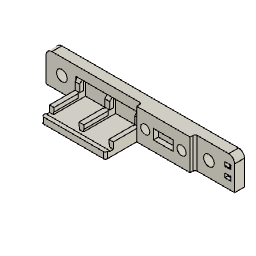
Bed WAGO Mount (Autodesk Fusion 360 design; units mm, degrees)
Autodesk Fusion 360 part; units mm, degrees
sketch "Sketch1" plane through (0, 0, 0) normal (0, 0, 1) x (1, 0, 0)
  line L0 (16.15, 6.1) -> (-16.15, 6.1)
  line L1 (-16.15, 6.1) -> (-16.15, -6.1)
  line L2 (-16.15, -6.1) -> (16.15, -6.1)
  line L3 (16.15, -6.1) -> (16.15, 6.1)
  line L4 (16.15, 6.1) -> (-16.15, -6.1) construction
  line L5 (-16.15, 6.1) -> (16.15, -6.1) construction
  dimension "d1" = 12.2
  dimension "d2" = 32.3
  constraint horizontal L0
  constraint perpendicular L0 L1
  constraint parallel L0 L2
  constraint parallel L1 L3
  constraint coincident L4 origin
  constraint coincident L5 origin
  measures "d1" distance of L0.start L2.end
  measures "d2" distance of L0.start L0.end
extrude "Extrude1" add sketch "Sketch1" along normal blind 22.25 makes body 1
sketch "Sketch2" plane through (0, 0, 22.25) normal (0, 0, 1) x (-1, 0, 0)
  line L0 (-16.15, 6.1) -> (-16.15, -6.1)
  line L1 (-16.15, -6.1) -> (16.15, -6.1)
  line L2 (16.15, -6.1) -> (16.15, 6.1)
  line L3 (16.15, 6.1) -> (-16.15, 6.1)
  line L4 (14.15, -6.1) -> (1, -6.1)
  line L5 (1, -6.1) -> (1, 4.1)
  line L6 (1, 4.1) -> (14.15, 4.1)
  line L7 (14.15, 4.1) -> (14.15, -6.1)
  line L8 (-1, -6.1) -> (-14.15, -6.1)
  line L9 (-14.15, -6.1) -> (-14.15, 4.1)
  line L10 (-14.15, 4.1) -> (-1, 4.1)
  line L11 (-1, 4.1) -> (-1, -6.1)
  dimension "d8" = 2
  dimension "d11" = 2
  dimension "d48" = 2
  dimension "d52" = 2
  constraint horizontal L4
  constraint vertical L5
  constraint horizontal L6
  constraint vertical L7
  constraint coincident L1 L4.start
  constraint horizontal L8
  constraint vertical L9
  constraint horizontal L10
  constraint vertical L11
  constraint coincident L1 L8.start
  constraint equal L6 L10
  constraint equal L5 L11
  measures "d8" distance of L4.end L8.start
  measures "d11" distance of L3 L9.end
  measures "d48" distance of L1.end L4.start
  measures "d52" distance of L0.end L8.end
extrude "Extrude2" cut sketch "Sketch2" against normal blind 20.25 contours L1 L8 L9 L10 L11 | L1 L4 L5 L6 L7 bodies 1
sketch "Sketch3" plane through (0, 0, 2) normal (0, 0, 1) x (-1, 0, 0)
  line L0 (-1, 4.1) -> (-14.15, 4.1)
  line L1 (-14.15, -6.1) -> (-1, -6.1)
  line L2 (-1, -6.1) -> (-1, 4.1)
  line L3 (14.15, 4.1) -> (1, 4.1)
  line L4 (1, 4.1) -> (1, -6.1)
  line L5 (1, -6.1) -> (14.15, -6.1)
  line L6 (14.15, -6.1) -> (14.15, 4.1)
  line L7 (-14.15, -6.1) -> (-1, -6.1)
  line L8 (-1, -6.1) -> (-14.15, -6.1)
  line L9 (-14.15, -6.1) -> (-14.15, -4.1)
  line L10 (-14.15, -4.1) -> (-1, -4.1)
  line L11 (-1, -4.1) -> (-1, -6.1)
  line L12 (-1, 4.1) -> (-14.15, 4.1)
  line L13 (-1, -6.1) -> (-1, 4.1)
  line L14 (14.15, 4.1) -> (1, 4.1)
  line L15 (1, 4.1) -> (1, -6.1)
  line L16 (1, -6.1) -> (14.15, -6.1)
  line L17 (14.15, -6.1) -> (14.15, 4.1)
  line L18 (1, -4.1) -> (14.15, -4.1)
  line L19 (-14.15, 4.1) -> (-14.15, -6.1)
  line L20 (-14.15, 4.1) -> (-14.15, -6.1)
  dimension "d12" = 2
  constraint horizontal L8
  constraint vertical L9
  constraint horizontal L10
  constraint vertical L11
  constraint coincident L1.end L2.start
  constraint coincident L15 L18.start
  constraint coincident L17 L18.end
  constraint perpendicular L17 L18
  constraint collinear L10 L18
  constraint coincident L1.start L7.start
  measures "d12" distance of L1.start L9.end
extrude "Extrude3" add sketch "Sketch3" along normal blind 2 contours L1 L2 L7 L8 L9 L10 L11 L13 L19 L20 | L4 L5 L6 L15 L16 L17 L18 bodies 1
sketch "Sketch4" plane through (0, 0, 22.25) normal (0, 0, 1) x (-1, 0, 0)
  line L0 (-1, 4.1) -> (-1, -6.1)
  line L1 (-1, -6.1) -> (1, -6.1)
  line L2 (1, -6.1) -> (1, 4.1)
  line L3 (1, 4.1) -> (14.15, 4.1)
  line L4 (14.15, 4.1) -> (14.15, -6.1)
  line L5 (14.15, -6.1) -> (16.15, -6.1)
  line L6 (16.15, -6.1) -> (16.15, 6.1)
  line L7 (16.15, 6.1) -> (-16.15, 6.1)
  line L8 (-16.15, 6.1) -> (-16.15, -6.1)
  line L9 (-14.15, 4.1) -> (-1, 4.1)
  line L10 (16.15, 4.1) -> (-16.15, 4.1)
  line L11 (-16.15, -6.1) -> (-14.15, -6.1)
  line L12 (-14.15, -6.1) -> (-14.15, 4.1)
  constraint coincident L6 L10.start
  constraint coincident L8 L10.end
  constraint perpendicular L8 L10
extrude "Extrude4" cut sketch "Sketch4" against normal blind 4 contours L0 L1 L2 L10 | L8 L10 L11 L12 | L4 L5 L6 L10 bodies 1
sketch "Sketch5" plane through (0, 0, 18.25) normal (0, 0, 1) x (-1, 0, 0)
  line L0 (16.15, 4.1) -> (14.15, 4.1)
  line L1 (14.15, 4.1) -> (14.15, -6.1)
  line L2 (-14.15, 4.1) -> (-16.15, 4.1)
  line L3 (-16.15, 4.1) -> (-16.15, -6.1)
  line L4 (-16.15, -6.1) -> (-14.15, -6.1)
  line L5 (1, -6.1) -> (1, 4.1)
  line L6 (1, 4.1) -> (-1, 4.1)
  line L7 (-1, 4.1) -> (-1, -6.1)
  line L8 (-1, -6.1) -> (1, -6.1)
  line L9 (16.15, 4.1) -> (14.15, 4.1)
  line L10 (16.15, -6.1) -> (16.15, 4.1)
  line L11 (16.15, -6.1) -> (-16.15, -6.1)
  line L12 (-16.15, -6.1) -> (-16.15, 0.85)
  line L13 (-16.15, 0.85) -> (16.15, 0.85)
  line L14 (16.15, 0.85) -> (16.15, -6.1)
  line L15 (16.15, -6.1) -> (16.15, 4.1)
  line L16 (14.15, 4.1) -> (14.15, -6.1)
  line L17 (14.15, -6.1) -> (16.15, -6.1)
  line L18 (14.15, -6.1) -> (16.15, -6.1)
  line L19 (-14.15, -6.1) -> (-14.15, 4.1)
  dimension "d17" = 3.25
  constraint horizontal L11
  constraint vertical L12
  constraint horizontal L13
  constraint vertical L14
  constraint coincident L3 L12.end
  constraint coincident L3.end L4.start
  constraint coincident L10.start L11.start
  measures "d17" distance of L2.end L12.end
extrude "Extrude5" cut sketch "Sketch5" against normal blind 13 contours L1 L10 L11 L13 L14 L15 L16 L17 L18 | L1 L5 L11 L13 L16 | L5 L7 L8 L11 L13 | L7 L11 L13 L19 | L3 L4 L11 L12 L13 L19 bodies 1
sketch "Sketch6" plane through (0, 0, 22.25) normal (0, 0, 1) x (-1, 0, 0)
  line L0 (-16.15, 4.1) -> (16.15, 4.1)
  line L1 (16.15, 4.1) -> (16.15, 6.1)
  line L2 (16.15, 6.1) -> (-16.15, 6.1)
  line L3 (-16.15, 6.1) -> (-16.15, 4.1)
  line L4 (16.15, 6.1) -> (-16.15, 6.1)
  line L5 (-16.15, 6.1) -> (-16.15, 3.6)
  line L6 (-16.15, 3.6) -> (16.15, 3.6)
  line L7 (16.15, 3.6) -> (16.15, 6.1)
  dimension "d20" = 2.5
  constraint horizontal L4
  constraint vertical L5
  constraint horizontal L6
  constraint vertical L7
  constraint coincident L1.end L2.start
  constraint collinear L3 L5
  measures "d20" distance of L2.end L5.end
extrude "Extrude6" add sketch "Sketch6" against normal blind 2 contours L0 L5 L6 L7 bodies 1
sketch "Sketch7" plane through (0, 0, 18.25) normal (0, 0, 1) x (-1, 0, 0)
  line L0 (16.15, 4.1) -> (14.15, 4.1)
  line L1 (14.15, 4.1) -> (14.15, 0.85) construction
  line L2 (13.9, 2.85) -> (16.15, 2.85)
  line L3 (1.25, 0.85) -> (-1.25, 0.85)
  line L4 (-1.25, 0.85) -> (-1.25, 2.85)
  line L5 (-1.25, 2.85) -> (1.25, 2.85)
  line L6 (1.25, 2.85) -> (1.25, 0.85)
  line L7 (16.15, 0.85) -> (13.9, 0.85)
  line L8 (13.9, 0.85) -> (13.9, 2.85)
  line L9 (13.9, 2.85) -> (16.15, 2.85)
  line L10 (16.15, 2.85) -> (16.15, 0.85)
  line L11 (-13.9, 0.85) -> (-16.15, 0.85)
  line L12 (-16.15, 0.85) -> (-16.15, 2.85)
  line L13 (-16.15, 2.85) -> (-13.9, 2.85)
  line L14 (-13.9, 2.85) -> (-13.9, 0.85)
  line L15 (16.15, 0.85) -> (16.15, 4.1)
  line L16 (16.15, 4.1) -> (14.15, 4.1)
  line L17 (1, 0.85) -> (1, 4.1) construction
  line L18 (1, 4.1) -> (-1, 4.1)
  line L19 (-1, 4.1) -> (-1, 0.85) construction
  line L20 (-16.15, 0.85) -> (-14.15, 0.85)
  line L21 (-14.15, 4.1) -> (-16.15, 4.1)
  line L22 (-16.15, 4.1) -> (-16.15, 0.85)
  line L23 (16.15, 0.85) -> (16.15, 4.1)
  line L24 (14.15, 4.1) -> (14.15, 0.85)
  line L25 (14.15, 0.85) -> (16.15, 0.85)
  line L26 (14.15, 0.85) -> (16.15, 0.85)
  line L27 (-1, 0.85) -> (1, 0.85)
  line L28 (-14.15, 0.85) -> (-14.15, 4.1)
  dimension "d23" = 2.25
  dimension "d50" = 2
  dimension "d51" = 2.5
  constraint horizontal L2
  constraint horizontal L3
  constraint vertical L4
  constraint horizontal L5
  constraint vertical L6
  constraint horizontal L7
  constraint vertical L8
  constraint horizontal L9
  constraint vertical L10
  constraint horizontal L11
  constraint vertical L12
  constraint horizontal L13
  constraint vertical L14
  constraint equal L7 L11
  constraint equal L4 L14
  constraint coincident L7.start L10.end
  constraint coincident L11.end L12.start
  constraint equal L6 L8
  measures "d23" distance of L7.start L7.end
  measures "d50" distance of L3.start L5.end
  measures "d51" distance of L3.start L3.end
extrude "Extrude7" add sketch "Sketch7" against normal blind 12.25 contours L2 L7 L9 L10 L15 L23 L24 L25 L26 | L2 L7 L8 L9 L24 | L3 L4 L5 L6 L27 | L11 L13 L14 L28 | L11 L12 L13 L20 L22 L28 bodies 1
sketch "Sketch8" plane through (0, 0, 5.25) normal (0, 0, 1) x (-1, 0, 0)
  line L0 (14.15, -6.1) -> (16.15, -6.1) construction
  line L1 (14.15, -6.1) -> (16.15, -6.1) construction
  line L2 (-14.15, 0.85) -> (-16.15, 0.85) construction
  line L3 (-16.15, 0.85) -> (-16.15, -6.1) construction
  line L4 (-16.15, -6.1) -> (-14.15, -6.1) construction
  line L5 (-1, -6.1) -> (-1, -4.1) construction
  line L6 (-1, -4.1) -> (-14.15, -4.1) construction
  line L7 (-14.15, -6.1) -> (-1, -6.1) construction
  line L8 (16.15, -6.1) -> (-16.15, -6.1)
  line L9 (-16.15, -6.1) -> (-16.15, -4.1)
  line L10 (-16.15, -4.1) -> (16.15, -4.1)
  line L11 (16.15, -4.1) -> (16.15, -6.1)
  line L12 (16.15, 0.85) -> (14.15, 0.85)
  line L13 (16.15, 0.85) -> (14.15, 0.85)
  line L14 (14.15, 0.85) -> (14.15, -6.1)
  line L15 (16.15, -6.1) -> (16.15, 0.85)
  line L16 (14.15, 0.85) -> (14.15, -6.1)
  line L17 (16.15, -6.1) -> (16.15, 0.85)
  line L18 (-14.15, -6.1) -> (-14.15, 0.85)
  line L19 (-14.15, -4.1) -> (-14.15, -6.1)
  constraint horizontal L8
  constraint vertical L9
  constraint horizontal L10
  constraint vertical L11
  constraint coincident L3 L9.end
  constraint coincident L0.end L1.end
  constraint coincident L6.end L10
extrude "Extrude8" cut sketch "Sketch8" against normal up to surface (1.25 mm away) contours L8 L10 L11 L14 L15 L16 L17 | L8 L10 L14 L16 L18 L19 | L8 L9 L10 L18 L19 bodies 1
sketch "Sketch9" plane through (0, 0, 5.25) normal (0, 0, 1) x (-1, 0, 0)
  line L0 (14.15, -4.1) -> (16.15, -4.1)
  line L1 (-16.15, -6.1) -> (16.15, -6.1)
  line L2 (16.15, -4.1) -> (14.15, -4.1)
  line L3 (-1, -4.1) -> (-14.15, -4.1)
  line L4 (16.15, -4.1) -> (13.9, -4.1)
  line L5 (13.9, -4.1) -> (13.9, 0.85)
  line L6 (13.9, 0.85) -> (16.15, 0.85)
  line L7 (16.15, 0.85) -> (16.15, -4.1)
  line L8 (1.25, -4.1044) -> (-1.25, -4.1044)
  line L9 (-1.25, -4.1044) -> (-1.25, 0.85)
  line L10 (-1.25, 0.85) -> (1.25, 0.85)
  line L11 (1.25, 0.85) -> (1.25, -4.1044)
  line L12 (-16.15, -4.1) -> (-13.9, -4.1)
  line L13 (-13.9, -4.1) -> (-13.9, 0.8544)
  line L14 (-13.9, 0.8544) -> (-16.15, 0.8544)
  line L15 (-16.15, 0.8544) -> (-16.15, -4.1)
  line L16 (16.15, 4.1) -> (14.15, 4.1)
  line L17 (14.15, 4.1) -> (14.15, 2.85)
  line L18 (13.9, 0.85) -> (16.15, 0.85)
  line L19 (14.15, -4.1) -> (1, -4.1)
  line L20 (16.15, 0.85) -> (16.15, 4.1)
  line L21 (14.15, 2.85) -> (13.9, 2.85)
  line L22 (13.9, 2.85) -> (13.9, 0.85)
  line L23 (1, 4.1) -> (-1, 4.1)
  line L24 (-1, 4.1) -> (-1, 2.85)
  line L25 (-1, 2.85) -> (-1.25, 2.85)
  line L26 (-1.25, 2.85) -> (-1.25, 0.85)
  line L27 (-1.25, 0.85) -> (1.25, 0.85)
  line L28 (1.25, 0.85) -> (1.25, 2.85)
  line L29 (16.15, 0.85) -> (14.15, 0.85)
  line L30 (13.9, 0.85) -> (16.15, 0.85)
  line L31 (16.15, -4.1) -> (16.15, 0.85)
  line L32 (14.15, 0.85) -> (14.15, -4.1)
  line L33 (16.15, -6.1) -> (16.15, -4.1)
  line L34 (1, -4.1) -> (-1, -4.1)
  line L35 (-14.15, -4.1) -> (-16.15, -4.1)
  line L36 (-16.15, -4.1) -> (-16.15, -6.1)
  line L37 (1, 2.85) -> (1, 4.1)
  line L38 (1.25, 2.85) -> (1, 2.85)
  line L39 (-14.15, 2.85) -> (-14.15, 4.1)
  line L40 (-14.15, 4.1) -> (-16.15, 4.1)
  line L41 (-16.15, 4.1) -> (-16.15, 0.85)
  line L42 (-16.15, 0.85) -> (-13.9, 0.85)
  line L43 (-13.9, 0.85) -> (-13.9, 2.85)
  line L44 (-13.9, 2.85) -> (-14.15, 2.85)
  constraint horizontal L4
  constraint vertical L5
  constraint horizontal L6
  constraint vertical L7
  constraint coincident L0.end L2.start
  constraint horizontal L8
  constraint vertical L9
  constraint horizontal L10
  constraint vertical L11
  constraint horizontal L12
  constraint vertical L13
  constraint horizontal L14
  constraint vertical L15
  constraint equal L9 L13
  constraint equal L6 L14
  constraint equal L6 L18
  constraint coincident L5.end L6.start
  constraint coincident L10.end L11.start
  constraint coincident L12.start L15.end
  constraint coincident L9.end L10.start
extrude "Extrude9" add sketch "Sketch9" against normal blind 2 contours L0 L2 L4 L6 L7 L18 L29 L30 L31 L32 | L4 L5 L6 L18 L19 L30 L32 | L3 L9 L10 L11 L19 L27 L34 | L3 L8 L9 L11 L19 L34 | L3 L12 L13 L15 L35 L42 | L13 L14 L15 L41 L42 L43 bodies 1
chamfer "Chamfer1" distance 1.25 angle 45 5 edges at (-15.025, 4.1, 5.25) (-15.025, 4.1, 5.25) (15.025, 4.1, 5.25) (0, 4.1044, 5.25) (15.025, 4.1, 5.25) on bodies 1
move_body "Move1" bodies 1 to x (1, 0, 0) y (0, 0, 1) z (0, -1, 0) at (0, 0, 0)
extrude "Extrude22" add 1 faces at (-5.3833, -7.4167, -6.1) along direction (0, 0, -1) blind 1 on bodies 1 bodies 1
sketch "Sketch10" plane through (0, 0, 0) normal (0, 1, 0) x (-1, 0, 0)
  line L0 (42.15, -7.1) -> (58.15, -7.1)
  line L1 (58.15, -7.1) -> (58.15, 8.9)
  line L2 (58.15, 8.9) -> (42.15, 8.9)
  line L3 (42.15, 8.9) -> (42.15, -7.1)
  line L4 (-16.15, -7.1) -> (-32.15, -7.1)
  line L5 (-32.15, -7.1) -> (-32.15, 8.9)
  line L6 (-32.15, 8.9) -> (-16.15, 8.9)
  line L7 (-16.15, 8.9) -> (-16.15, -7.1)
  line L8 (42.15, 8.9) -> (58.15, -7.1) construction
  line L9 (-32.15, -7.1) -> (-16.15, 8.9) construction
  circle A0 centre (50.15, 0.9) radius 2.7
  circle A1 centre (-24.15, 0.9) radius 2.7
  line L10 (-16.15, 6.1) -> (-16.15, -7.1)
  line L11 (16.15, -7.1) -> (16.15, 6.1)
  line L12 (16.15, 6.1) -> (-16.15, 6.1)
  line L13 (16.15, -7.1) -> (42.15, -7.1)
  line L14 (42.15, 8.9) -> (-16.15, 8.9)
  line L15 (-16.15, -7.1) -> (16.15, -7.1)
  dimension "d35" = 5.4
  dimension "d55" = 16
  dimension "d72" = 26
  constraint horizontal L0
  constraint vertical L1
  constraint horizontal L2
  constraint vertical L3
  constraint horizontal L4
  constraint vertical L5
  constraint horizontal L6
  constraint vertical L7
  constraint equal L1 L5
  constraint equal L1 L2
  constraint equal L5 L6
  constraint midpoint L8 A0.centre
  constraint midpoint L9 A1.centre
  constraint equal A0 A1
  constraint coincident L4.start L7.end
  constraint coincident L11.start L13.start
  constraint perpendicular L11 L13
  constraint coincident L0.start L3.end
  measures "d35" diameter of A0
  measures "d55" distance of L0.end L1.end
  measures "d72" distance of L11.start L0.start
extrude "Extrude10" add sketch "Sketch10" against normal blind 4 contours L0 L1 L2 L3 | L3 L7 L11 L12 L13 L14 | L4 L5 L6 L7 L10 bodies 1
extrude "Extrude17" add 1 faces at (-1.0667, 0, -5.2128) along direction (0, 1, 0) blind 1 on bodies 1 bodies 1
sketch "Sketch19" plane through (0, -4, 0) normal (0, -1, 0) x (1, 0, 0)
  line L0 (-29.65, 4.9) -> (-29.65, -3.1) construction
  line L1 (-38.85, 0.9) -> (-20.45, 0.9) construction
  circle A0 centre (-38.85, 0.9) radius 2.3
  circle A1 centre (-20.45, 0.9) radius 2.3
  circle A2 centre (24.15, 0.9) radius 2.7
  circle A3 centre (-50.15, 0.9) radius 2.7
  line L2 (-1.25, 4.1) -> (-1.25, 4.1044)
  line L3 (-1.25, 4.1044) -> (1.25, 4.1044)
  line L4 (1.25, 4.1044) -> (1.25, 4.1)
  line L5 (1.25, 4.1) -> (13.9, 4.1)
  line L6 (13.9, 4.1) -> (16.15, 4.1)
  line L7 (16.15, 4.1) -> (16.15, -7.1)
  line L8 (16.15, -7.1) -> (32.15, -7.1)
  line L9 (32.15, -7.1) -> (32.15, 8.9)
  line L10 (32.15, 8.9) -> (-58.15, 8.9)
  line L11 (-58.15, 8.9) -> (-58.15, -7.1)
  line L12 (-58.15, -7.1) -> (-16.15, -7.1)
  line L13 (-16.15, -7.1) -> (-16.15, 4.1)
  line L14 (-16.15, 4.1) -> (-13.9, 4.1)
  line L15 (-13.9, 4.1) -> (-1.25, 4.1)
  line L16 (-42.15, 4.9) -> (-17.15, 4.9) construction
  line L17 (-17.15, 4.9) -> (-17.15, -3.1) construction
  line L18 (-17.15, -3.1) -> (-42.15, -3.1) construction
  line L19 (-42.15, -3.1) -> (-42.15, 4.9) construction
  line L20 (-42.15, 0.9) -> (-58.15, 0.9) construction
  dimension "d91" = 18.4
  dimension "d92" = 4.6
  dimension "d93" = 4.6
  dimension "d97" = 8
  dimension "d98" = 25
  dimension "d108" = 1
  constraint horizontal L1
  constraint midpoint L0 L1
  constraint coincident L1.start A0.centre
  constraint coincident L1.end A1.centre
  constraint horizontal L16
  constraint vertical L17
  constraint horizontal L18
  constraint vertical L19
  constraint midpoint L19 L20.start
  constraint perpendicular L19 L20
  constraint midpoint L11 L20.end
  constraint midpoint L0.start L16
  constraint midpoint L0.end L18
  measures "d91" distance of L1.start L1.end
  measures "d92" diameter of A0
  measures "d93" diameter of A1
  measures "d97" distance of L16.start L18.end
  measures "d98" distance of L16.start L16.end
  measures "d108" distance of L13 L17
extrude "Extrude20" cut sketch "Sketch19" against normal blind 4 contours A0 | A1 bodies 1
sketch "Sketch21" plane through (0, -4, 0) normal (0, -1, 0) x (1, 0, 0)
  circle A0 centre (-20.45, 0.9) radius 2.3
  circle A1 centre (-38.85, 0.9) radius 2.3
  circle A2 centre (24.15, 0.9) radius 2.7
  circle A3 centre (-50.15, 0.9) radius 2.7
  line L0 (-1.25, 4.1) -> (-1.25, 4.1044)
  line L1 (-1.25, 4.1044) -> (1.25, 4.1044)
  line L2 (1.25, 4.1044) -> (1.25, 4.1)
  line L3 (1.25, 4.1) -> (13.9, 4.1)
  line L4 (13.9, 4.1) -> (16.15, 4.1)
  line L5 (16.15, 4.1) -> (16.15, -7.1)
  line L6 (16.15, -7.1) -> (32.15, -7.1)
  line L7 (32.15, -7.1) -> (32.15, 8.9)
  line L8 (32.15, 8.9) -> (-58.15, 8.9)
  line L9 (-58.15, 8.9) -> (-58.15, -7.1)
  line L10 (-58.15, -7.1) -> (-16.15, -7.1)
  line L11 (-16.15, -7.1) -> (-16.15, 4.1)
  line L12 (-16.15, 4.1) -> (-13.9, 4.1)
  line L13 (-13.9, 4.1) -> (-1.25, 4.1)
  line L14 (-34.65, 3.4) -> (-24.65, 3.4)
  line L15 (-24.65, 3.4) -> (-24.65, -1.6)
  line L16 (-24.65, -1.6) -> (-34.65, -1.6)
  line L17 (-34.65, -1.6) -> (-34.65, 3.4)
  line L18 (-38.85, 0.9) -> (-34.65, 0.9) construction
  line L19 (-24.65, 0.9) -> (-20.45, 0.9) construction
  dimension "d99" = 10
  dimension "d100" = 5
  constraint horizontal L14
  constraint vertical L15
  constraint horizontal L16
  constraint vertical L17
  constraint coincident A1.centre L18.start
  constraint perpendicular L17 L18
  constraint midpoint L17 L18.end
  constraint midpoint L15 L19.start
  constraint perpendicular L15 L19
  constraint coincident A0.centre L19.end
  constraint equal L18 L19
  measures "d99" distance of L14.start L14.end
  measures "d100" distance of L14.start L16.end
extrude "Extrude21" cut sketch "Sketch21" against normal blind 2.5 contours L14 L15 L16 L17 bodies 1
sketch "Sketch11" plane through (0, -4, 0) normal (0, -1, 0) x (1, 0, 0)
  circle A0 centre (24.15, 0.9) radius 6
  circle A1 centre (-50.15, 0.9) radius 6
  circle A2 centre (24.15, 0.9) radius 2.7
  circle A3 centre (-50.15, 0.9) radius 2.7
  line L0 (-1.25, 4.1) -> (-1.25, 4.1044)
  line L1 (-1.25, 4.1044) -> (1.25, 4.1044)
  line L2 (1.25, 4.1044) -> (1.25, 4.1)
  line L3 (1.25, 4.1) -> (13.9, 4.1)
  line L4 (13.9, 4.1) -> (16.15, 4.1)
  line L5 (16.15, 4.1) -> (16.15, -7.1)
  line L6 (16.15, -7.1) -> (32.15, -7.1)
  line L7 (32.15, -7.1) -> (32.15, 8.9)
  line L8 (32.15, 8.9) -> (-58.15, 8.9)
  line L9 (-58.15, 8.9) -> (-58.15, -7.1)
  line L10 (-16.15, -7.1) -> (-16.15, 4.1)
  line L11 (-16.15, 4.1) -> (-13.9, 4.1)
  line L12 (-13.9, 4.1) -> (-1.25, 4.1)
  line L13 (-58.15, -7.1) -> (-16.15, -7.1)
  line L14 (-24.65, 3.4) -> (-24.65, -1.6)
  line L15 (-24.65, -1.6) -> (-34.65, -1.6)
  line L16 (-34.65, -1.6) -> (-34.65, 3.4)
  line L17 (-34.65, 3.4) -> (-24.65, 3.4)
  circle A4 centre (-20.45, 0.9) radius 2.3
  circle A5 centre (-38.85, 0.9) radius 2.3
  dimension "d38" = 12
  dimension "d39" = 12
  constraint coincident A0.centre A2.centre
  constraint coincident A1.centre A3.centre
  measures "d38" diameter of A0
  measures "d39" diameter of A1
extrude "Extrude11" [suppressed]
sketch "Sketch13" plane through (0, 1, 0) normal (0, 1, 0) x (-1, 0, 0)
  line L0 (33, 2.9) -> (-7, 2.9)
  line L1 (-7, 2.9) -> (-7, -1.1)
  line L2 (-7, -1.1) -> (33, -1.1)
  line L3 (33, -1.1) -> (33, 2.9)
  line L4 (-7, 0.9) -> (-24.15, 0.9) construction
  line L5 (33, 0.9) -> (50.15, 0.9) construction
  circle A0 centre (50.15, 0.9) radius 2.7
  circle A1 centre (-24.15, 0.9) radius 2.7
  dimension "d61" = 4
  dimension "d62" = 40
  constraint horizontal L0
  constraint perpendicular L0 L1
  constraint parallel L0 L2
  constraint parallel L1 L3
  constraint midpoint L1 L4.start
  constraint perpendicular L1 L4
  constraint midpoint L3 L5.start
  constraint perpendicular L3 L5
  constraint coincident L4.end A1.centre
  constraint coincident L5.end A0.centre
  constraint equal L4 L5
  measures "d61" distance of L0.start L2.end
  measures "d62" distance of L0.start L0.end
extrude "Extrude15" add sketch "Sketch13" along normal blind 0.8 contours L0 L1 L2 L3 bodies 1
sketch "Sketch22" plane through (0, -4, 0) normal (0, -1, 0) x (1, 0, 0)
  line L0 (-24.65, 3.4) -> (-24.65, -1.6)
  line L1 (-24.65, -1.6) -> (-34.65, -1.6)
  line L2 (-34.65, -1.6) -> (-34.65, 3.4)
  line L3 (-34.65, 3.4) -> (-24.65, 3.4)
  circle A0 centre (-20.45, 0.9) radius 2.3
  circle A1 centre (-38.85, 0.9) radius 2.3
  line L4 (-1.25, 4.1) -> (-1.25, 4.1044)
  line L5 (-1.25, 4.1044) -> (1.25, 4.1044)
  line L6 (1.25, 4.1044) -> (1.25, 4.1)
  line L7 (1.25, 4.1) -> (13.9, 4.1)
  line L8 (13.9, 4.1) -> (16.15, 4.1)
  line L9 (16.15, 4.1) -> (16.15, -7.1)
  line L10 (16.15, -7.1) -> (32.15, -7.1)
  line L11 (32.15, -7.1) -> (32.15, 8.9)
  line L12 (32.15, 8.9) -> (-58.15, 8.9)
  line L13 (-58.15, 8.9) -> (-58.15, -7.1)
  line L14 (-58.15, -7.1) -> (-16.15, -7.1)
  line L15 (-16.15, -7.1) -> (-16.15, 4.1)
  line L16 (-16.15, 4.1) -> (-13.9, 4.1)
  line L17 (-13.9, 4.1) -> (-1.25, 4.1)
  line L18 (-58.15, 8.9) -> (-63.15, 8.9)
  line L19 (-63.15, 8.9) -> (-63.15, -7.1)
  line L20 (-63.15, -7.1) -> (-58.15, -7.1)
  line L21 (-61.15, 4.4) -> (-58.15, 4.4)
  line L22 (-58.15, 4.4) -> (-58.15, 2.4)
  line L23 (-58.15, 2.4) -> (-61.15, 2.4)
  line L24 (-61.15, 2.4) -> (-61.15, 4.4)
  line L25 (-61.15, -0.6) -> (-58.15, -0.6)
  line L26 (-58.15, -0.6) -> (-58.15, -2.6)
  line L27 (-58.15, -2.6) -> (-61.15, -2.6)
  line L28 (-61.15, -2.6) -> (-61.15, -0.6)
  line L29 (-61.15, 2.4) -> (-61.15, -0.6) construction
  line L30 (-61.15, 0.9) -> (-63.15, 0.9) construction
  circle A2 centre (-50.15, 0.9) radius 2.7
  circle A3 centre (24.15, 0.9) radius 2.7
  dimension "d115" = 3
  dimension "d116" = 2
  dimension "d117" = 5
  dimension "d118" = 3
  constraint coincident L12.end L13.start
  constraint perpendicular L13 L18
  constraint perpendicular L14 L19
  constraint coincident L13.end L14.start
  constraint perpendicular L13 L20
  constraint horizontal L21
  constraint vertical L22
  constraint horizontal L23
  constraint vertical L24
  constraint horizontal L25
  constraint vertical L26
  constraint horizontal L27
  constraint vertical L28
  constraint equal L24 L28
  constraint equal L21 L25
  constraint perpendicular L23 L29
  constraint coincident L25.start L28.end
  constraint collinear L13 L22
  constraint midpoint L29 L30.start
  constraint perpendicular L29 L30
  constraint midpoint L19 L30.end
  measures "d115" distance of L21.start L21.end
  measures "d116" distance of L21.start L23.end
  measures "d117" distance of L12.end L18.end
  measures "d118" distance of L23.end L25.start
extrude "Extrude24" add sketch "Sketch22" against normal up to surface (5 mm away) contours L13 L18 L19 L20 L21 L23 L24 L25 L27 L28 bodies 1
sketch "Sketch23" plane through (0, 1, 0) normal (0, 1, 0) x (-1, 0, 0)
  line L0 (63.15, 8.9) -> (-32.15, 8.9)
  line L1 (-32.15, 8.9) -> (-32.15, -7.1)
  line L2 (-32.15, -7.1) -> (63.15, -7.1)
  line L3 (63.15, -7.1) -> (63.15, 8.9)
  line L4 (58.15, -2.6) -> (58.15, -0.6)
  line L5 (58.15, -0.6) -> (61.15, -0.6)
  line L6 (61.15, -0.6) -> (61.15, -2.6)
  line L7 (61.15, -2.6) -> (58.15, -2.6)
  line L8 (33, -1.1) -> (-7, -1.1)
  line L9 (-7, -1.1) -> (-7, 2.9)
  line L10 (-7, 2.9) -> (33, 2.9)
  line L11 (33, 2.9) -> (33, -1.1)
  circle A0 centre (50.15, 0.9) radius 2.7
  circle A1 centre (-24.15, 0.9) radius 2.7
  line L12 (58.15, 4.4) -> (61.15, 4.4)
  line L13 (61.15, 4.4) -> (61.15, 2.4)
  line L14 (61.15, 2.4) -> (58.15, 2.4)
  line L15 (58.15, 2.4) -> (58.15, 4.4)
  line L16 (58.15, 2.4) -> (58.15, -0.6)
  line L17 (61.15, 2.4) -> (61.15, -0.6)
  constraint coincident L14.end L15.start
  constraint coincident L4.end L5.start
  constraint coincident L13.end L14.start
  constraint coincident L5.end L6.start
extrude "Extrude25" cut sketch "Sketch23" against normal up to surface (4 mm away) contours L5 L14 L16 L17 bodies 1
sketch "Sketch24" plane through (0, 1, 0) normal (0, 1, 0) x (-1, 0, 0)
  line L0 (58.15, -2.6) -> (58.15, 4.4)
  line L1 (58.15, 4.4) -> (61.15, 4.4)
  line L2 (61.15, 4.4) -> (61.15, -2.6)
  line L3 (61.15, -2.6) -> (58.15, -2.6)
  line L4 (63.15, 8.9) -> (-32.15, 8.9)
  line L5 (-32.15, 8.9) -> (-32.15, -7.1)
  line L6 (-32.15, -7.1) -> (63.15, -7.1)
  line L7 (63.15, -7.1) -> (63.15, 8.9)
  line L8 (33, -1.1) -> (-7, -1.1)
  line L9 (-7, -1.1) -> (-7, 2.9)
  line L10 (-7, 2.9) -> (33, 2.9)
  line L11 (33, 2.9) -> (33, -1.1)
  circle A0 centre (50.15, 0.9) radius 2.7
  circle A1 centre (-24.15, 0.9) radius 2.7
extrude "Extrude26" add sketch "Sketch24" against normal up to surface (2.5 mm away) contours L0 L1 L2 L3 bodies 1
sketch "Sketch25" plane through (0, -4, 0) normal (0, -1, 0) x (1, 0, 0)
  line L0 (-58.15, 4.4) -> (-58.15, 2.4)
  line L1 (-58.15, 2.4) -> (-61.15, 2.4)
  line L2 (-61.15, 2.4) -> (-61.15, 4.4)
  line L3 (-61.15, 4.4) -> (-58.15, 4.4)
  line L4 (32.15, 8.9) -> (-63.15, 8.9)
  line L5 (-63.15, 8.9) -> (-63.15, -7.1)
  line L6 (-63.15, -7.1) -> (-16.15, -7.1)
  line L7 (-16.15, -7.1) -> (-16.15, 4.1)
  line L8 (-16.15, 4.1) -> (-13.9, 4.1)
  line L9 (-13.9, 4.1) -> (-1.25, 4.1)
  line L10 (-1.25, 4.1) -> (-1.25, 4.1044)
  line L11 (-1.25, 4.1044) -> (1.25, 4.1044)
  line L12 (1.25, 4.1044) -> (1.25, 4.1)
  line L13 (1.25, 4.1) -> (13.9, 4.1)
  line L14 (13.9, 4.1) -> (16.15, 4.1)
  line L15 (16.15, 4.1) -> (16.15, -7.1)
  line L16 (16.15, -7.1) -> (32.15, -7.1)
  line L17 (32.15, -7.1) -> (32.15, 8.9)
  line L18 (-24.65, 3.4) -> (-24.65, -1.6)
  line L19 (-24.65, -1.6) -> (-34.65, -1.6)
  line L20 (-34.65, -1.6) -> (-34.65, 3.4)
  line L21 (-34.65, 3.4) -> (-24.65, 3.4)
  circle A0 centre (-20.45, 0.9) radius 2.3
  circle A1 centre (-38.85, 0.9) radius 2.3
  line L22 (-58.15, -2.6) -> (-61.15, -2.6)
  line L23 (-61.15, -2.6) -> (-61.15, -0.6)
  line L24 (-61.15, -0.6) -> (-58.15, -0.6)
  line L25 (-58.15, -0.6) -> (-58.15, -2.6)
  line L26 (-43.15, 8.9) -> (-16.15, 8.9)
  line L27 (-16.15, 8.9) -> (-16.15, -7.1)
  line L28 (-16.15, -7.1) -> (-43.15, -7.1)
  line L29 (-43.15, -7.1) -> (-43.15, 8.9)
  circle A2 centre (-50.15, 0.9) radius 2.7
  circle A3 centre (24.15, 0.9) radius 2.7
  dimension "d131" = 27
  constraint horizontal L26
  constraint vertical L27
  constraint horizontal L28
  constraint vertical L29
  constraint coincident L6.end L7.start
  constraint coincident L4 L26.start
  measures "d131" distance of L26.start L26.end
extrude "Extrude27" add sketch "Sketch25" along normal blind 2.5 contours L4 L6 L7 L26 L27 L28 L29 bodies 1
extrude "Extrude28" add 1 faces at (-31.3167, -1.5, 0.0667) along direction (0, -1, 0) blind 2.5 on bodies 1 bodies 1
chamfer "Chamfer8" distance 1 angle 45 2 edges at (-59.65, -1.5, -2.6) (-59.65, -1.5, 4.4) on bodies 1
chamfer "Chamfer9" distance 0.6 angle 45 2 edges at (-59.65, -3, -0.6) (-59.65, -3, 2.4) on bodies 1
chamfer "Chamfer6" distance 0.8 angle 45 2 edges at (-13, 1, -1.1) (-13, 1, 2.9) on bodies 1
extrude "Extrude29" cut 2 faces at (-20.7301, 0, 1.2293) (-38.9073, 0, -0.7283) along direction (0, 1, 0) through all on bodies 1 bodies 1
fillet "Fillet3" radius 3 2 edges at (32.15, -1.5, 8.9) (-63.15, -1.5, 8.9) on bodies 1
fillet "Fillet4" radius 1 5 edges at (16.15, -4, -1.5) (-16.15, -22.25, -5.35) (16.15, -22.25, -5.35) (-16.15, -4, 6.5) (-43.15, -4, 0.9) on bodies 1
chamfer "Chamfer7" distance 0.4 angle 45 1 faces at (5.05, -11.25, -7.1) on bodies 1
mirror "Mirror1" about plane through (0, 0, 0) normal (1, 0, 0) of bodies 1 makes body 2
delete_body "RemoveBody1" bodies 1
